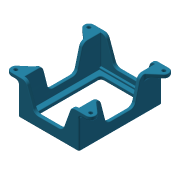
# Autodesk Inventor part: VatHolder
Saved by Autodesk Inventor 2014 (Build 180170000, 170)
## iProperties
Created: 2014-09-09
Part Number: VatHolder
Material: Generic
Document SubType Name: Modeling
Designer: Peele
Density: 1 g/cm^3
Appearance: Turquoise
Author: Peele
Autodesk Inventor part; units mm, degrees
ref_plane "YZ Plane" through (0, 0, 0) normal (1, 0, 0) x (0, 1, 0)
ref_plane "XZ Plane" through (0, 0, 0) normal (0, 1, 0) x (-1, 0, 0)
ref_plane "XY Plane" through (0, 0, 0) normal (0, 0, 1) x (1, 0, 0)
sketch "Sketch1" plane through (0, 0, 0) normal (0, 0, 1) x (1, 0, 0)
  line L0 (-38.1, -53.8) -> (38.1, -53.8)
  line L1 (38.1, -53.8) -> (38.1, 53.8)
  line L2 (38.1, 53.8) -> (-38.1, 53.8)
  line L3 (-38.1, 53.8) -> (-38.1, -53.8)
  line L4 (-38.1, -53.8) -> (38.1, 53.8) construction
  line L5 (38.1, -53.8) -> (-38.1, 53.8) construction
  line L6 (-30.6, -46.3) -> (30.6, -46.3)
  line L7 (30.6, -46.3) -> (30.6, 46.3)
  line L8 (30.6, 46.3) -> (-30.6, 46.3)
  line L9 (-30.6, 46.3) -> (-30.6, -46.3)
  line L10 (-30.6, -46.3) -> (30.6, 46.3) construction
  line L11 (30.6, -46.3) -> (-30.6, 46.3) construction
  line L12 (43.6, -59.3) -> (-43.6, -59.3)
  line L13 (-43.6, -59.3) -> (-43.6, 59.3)
  line L14 (-43.6, 59.3) -> (43.6, 59.3)
  line L15 (43.6, 59.3) -> (43.6, -59.3)
  line L16 (43.6, -59.3) -> (-43.6, 59.3) construction
  line L17 (-43.6, -59.3) -> (43.6, 59.3) construction
  point P0 (0, 0)
  dimension "d0" = 76.2
  dimension "d1" = 107.6
  dimension "d2" = 7.5
  dimension "d3" = 7.5
  dimension "d4" = 5.5
  dimension "d5" = 5.5
  constraints: 36 end point, 6 midpoint, 6 parallel, 3 horizontal, 3 perpendicular
  measures "d0" distance of L1.end L2.end
  measures "d1" distance of L0.end L1.end
  measures "d2" distance between parallel lines of L3 L9
  measures "d3" distance between parallel lines of L2 L8
  measures "d4" distance between parallel lines of L14 L2
  measures "d5" distance between parallel lines of L13 L3
extrude "Extrusion1" add sketch "Sketch1" along normal blind 5 contours L3 L2 L1 L0 | L12 L13 L14 L15
sketch "Sketch2" plane through (0, 0, 5) normal (0, 0, 1) x (1, 0, 0)
  line L0 (-43.6, 59.3) -> (-43.6, -59.3) projected
  line L1 (43.6, -59.3) -> (-43.6, -59.3)
  line L2 (-43.6, -59.3) -> (-43.6, 59.3)
  line L3 (-43.6, 59.3) -> (43.6, 59.3)
  line L4 (43.6, 59.3) -> (43.6, -59.3)
  line L5 (43.6, -59.3) -> (-43.6, 59.3) construction
  line L6 (-43.6, -59.3) -> (43.6, 59.3) construction
  line L7 (38.6, -54.3) -> (-38.6, -54.3)
  line L8 (-38.6, -54.3) -> (-38.6, 54.3)
  line L9 (-38.6, 54.3) -> (38.6, 54.3)
  line L10 (38.6, 54.3) -> (38.6, -54.3)
  line L11 (38.6, -54.3) -> (-38.6, 54.3) construction
  line L12 (-38.6, -54.3) -> (38.6, 54.3) construction
  point P0 (0, 0)
  dimension "d8" = 5
  dimension "d9" = 5
  constraints: 24 end point, 4 midpoint, 4 parallel, 2 horizontal, 2 perpendicular
  measures "d8" distance between parallel lines of L3 L9
  measures "d9" distance between parallel lines of L0 L8
extrude "Extrusion2" add sketch "Sketch2" along normal blind 45
sketch "Sketch3" plane through (-43.6, -59.3, 0) normal (0, -1, 0) x (1, 0, 0)
  line L0 (87.2, 0) -> (0, 0) projected
  line L1 (0, 50) -> (87.2, 50) projected
  line L2 (0, 0) -> (0, 50) projected
  line L3 (11.1, 50) -> (23.6, 15)
  line L4 (23.6, 15) -> (63.6, 15)
  line L5 (63.6, 15) -> (76.1, 50)
  line L6 (11.1, 50) -> (76.1, 50)
  line L7 (43.6, 0) -> (43.6, 15) construction
  dimension "d12" = 40
  dimension "d13" = 15
  dimension "d14" = 65
  constraints: 10 end point, 2 point on line, 1 collinear, 1 equal length, 1 midpoint, 1 perpendicular, 1 vertical
  measures "d12" distance of L3.end L4.end
  measures "d13" distance between parallel lines of L0 L4
  measures "d14" distance of L5.end L3.start
extrude "Extrusion3" cut sketch "Sketch3" against normal through all
sketch "Sketch4" plane through (0, 0, 50) normal (0, 0, 1) x (1, 0, 0)
  line L0 (43.6, -59.3) -> (43.6, 59.3) projected
  line L1 (43.6, -59.3) -> (43.6, -34.3)
  line L2 (43.6, -59.3) -> (53.6, -59.3)
  line L3 (58.199, -47.0228) -> (43.6, -34.3)
  arc A0 (53.6, -59.3) -> (58.199, -47.0228) centre (53.6, -52.3) ccw
  circle A1 centre (53.6, -52.3) radius 2.25
  point P0 (0, 0)
  dimension "d17" = 4.5
  dimension "d18" = 10
  dimension "d19" = 7
  dimension "d20" = 25
  constraints: 6 end point, 2 centre point, 2 point on circle, 2 tangent, 1 coincident, 1 perpendicular, 1 point on line
  measures "d17" diameter of A1
  measures "d18" distance from line of A0.centre L0
  measures "d19" distance from line of A0.centre L2
  measures "d20" distance from line of L1.end L2
extrude "Extrusion4" add sketch "Sketch4" against normal blind 6
mirror "Mirror1" about plane through (0, 0, 0) normal (0, 1, 0) of "Extrusion4"
mirror "Mirror2" about plane through (0, 0, 0) normal (1, 0, 0) of "Extrusion4", "Mirror1"
sketch "Sketch5" plane through (43.6, -59.3, 0) normal (1, 0, 0) x (0, 0, -1)
  line L0 (0, 118.6) -> (-44, 118.6) projected
  line L1 (-15, 79.3) -> (-15, 39.3)
  line L2 (-50, 93.6) -> (-50, 25)
  line L3 (-15, 39.3) -> (-50, 30.3)
  line L4 (-15, 79.3) -> (-50, 88.3)
  line L5 (-50, 30.3) -> (-50, 88.3)
  line L6 (0, 0) -> (-15, 39.3) construction
  line L7 (-15, 79.3) -> (0, 118.6) construction
  point P0 (0, 59.3)
  point P1 (-15, 118.6)
  dimension "d23" = 40
  dimension "d24" = 58
  constraints: 14 end point, 3 point on line, 2 equal length, 1 collinear, 1 perpendicular
  measures "d23" distance of L1.end L1.start
  measures "d24" distance of L3.end L4.end
extrude "Extrusion5" cut sketch "Sketch5" against normal through all
sketch "Sketch6" plane through (0, 0, 5) normal (0, 0, 1) x (1, 0, 0)
  line L0 (-38.6, 54.3) -> (-38.6, -54.3) projected
  line L1 (-38.6, -54.3) -> (38.6, -54.3) projected
  line L2 (38.6, -54.3) -> (38.6, 54.3) projected
  line L3 (-38.6, 54.3) -> (38.6, 54.3)
  line L4 (38.6, 54.3) -> (38.6, 51.8)
  line L5 (38.6, 51.8) -> (-38.6, 51.8)
  line L6 (-38.6, 51.8) -> (-38.6, 54.3)
  line L7 (38.6, -54.3) -> (-38.6, -54.3)
  line L8 (-38.6, -54.3) -> (-38.6, -51.8)
  line L9 (-38.6, -51.8) -> (38.6, -51.8)
  line L10 (38.6, -51.8) -> (38.6, -54.3)
  point P0 (0, 0)
  dimension "d27" = 2.5
  dimension "d28" = 2.5
  constraints: 16 end point, 4 parallel, 2 horizontal, 2 perpendicular, 2 point on line
  measures "d27" distance of L5.end L0.start
  measures "d28" distance between parallel lines of L1 L9
extrude "Extrusion6" add sketch "Sketch6" along normal blind 2.9 contours L3 L2 L5 L0 | L9 L2 L1 L0
fillet "Fillet1" radius 8 16 edges at (-20, -56.8, 15) (-32.5, -56.8, 50) (-41.1, -29, 50) (-41.1, -20, 15) (-41.1, 29, 50) (-41.1, 20, 15) (-20, 56.8, 15) (-32.5, 56.8, 50) (20, 56.8, 15) (32.5, 56.8, 50) (41.1, 29, 50) (41.1, 20, 15) (20, -56.8, 15) (32.5, -56.8, 50) (41.1, -29, 50) (41.1, -20, 15)
fillet "Fillet2" radius 4 12 edges at (-43.6, -46.8, 44) (-43.6, -34.3, 46.9744) (-43.6, 46.8, 44) (-43.6, 34.3, 46.9744) (30.6, 46.3, 2.5) (-30.6, 46.3, 2.5) (-30.6, -46.3, 2.5) (30.6, -46.3, 2.5) (43.6, -34.3, 46.9744) (43.6, -46.8, 44) (43.6, 46.8, 44) (43.6, 34.3, 46.9744)
fillet "Fillet3" radius 1 18 edges at (0, -51.8, 7.9) (-29.4284, -45.1284, 5) (-30.6, 0, 5) (-29.4284, 45.1284, 5) (0, 46.3, 5) (29.4284, 45.1284, 5) (30.6, 0, 5) (29.4284, -45.1284, 5) (0, -46.3, 5) (29.4284, -45.1284, 0) (30.6, 0, 0) (29.4284, 45.1284, 0) (0, 46.3, 0) (-29.4284, 45.1284, 0) (-30.6, 0, 0) (-29.4284, -45.1284, 0) (0, -46.3, 0) (0, 51.8, 7.9)
fillet "Fillet4" radius 1 36 edges at (38.6, -30.301, 48.3221) (38.6, -24.5, 32.5) (38.6, -18.699, 16.6779) (38.6, 0, 15) (38.6, 18.699, 16.6779) (38.6, 24.5, 32.5) (38.6, 30.301, 48.3221) (38.6, 44.7516, 50) (38.6, -44.7516, 50) (26.25, -54.3, 32.5) (18.9706, -54.3, 16.4607) (0, -54.3, 15) (-18.9706, -54.3, 16.4607) (-26.25, -54.3, 32.5) (-33.5294, -54.3, 48.5393) (-38.3689, -54.3, 50) (38.3689, -54.3, 50) (33.5294, -54.3, 48.5393) (38.3689, 54.3, 50) (26.25, 54.3, 32.5) (18.9706, 54.3, 16.4607) (0, 54.3, 15) (-18.9706, 54.3, 16.4607) (-26.25, 54.3, 32.5) (-33.5294, 54.3, 48.5393) (-38.3689, 54.3, 50) (33.5294, 54.3, 48.5393) (-38.6, 30.301, 48.3221) (-38.6, 24.5, 32.5) (-38.6, 18.699, 16.6779) (-38.6, 0, 15) (-38.6, -18.699, 16.6779) (-38.6, -24.5, 32.5) (-38.6, -30.301, 48.3221) (-38.6, -44.7516, 50) (-38.6, 44.7516, 50)
fillet "Fillet5" radius 1 48 edges at (60.1552, 54.7555, 50) (51.5855, 41.2592, 50) (44.8171, 35.3534, 50) (43.8895, 33.9741, 49.905) (43.6, 29.2824, 47.38) (43.6, 24.5, 32.5) (43.6, 18.699, 16.6779) (43.6, 0, 15) (43.6, -18.699, 16.6779) (43.6, -24.5, 32.5) (43.6, -29.2824, 47.38) (43.8895, -33.9741, 49.905) (44.8171, -35.3534, 50) (51.5855, -41.2592, 50) (60.1552, -54.7555, 50) (45.8689, -59.3, 50) (33.5294, -59.3, 48.5393) (26.25, -59.3, 32.5) (18.9706, -59.3, 16.4607) (0, -59.3, 15) (-18.9706, -59.3, 16.4607) (-26.25, -59.3, 32.5) (-33.5294, -59.3, 48.5393) (-45.8689, -59.3, 50) (-60.1552, -54.7555, 50) (-51.5855, -41.2592, 50) (-44.8171, -35.3534, 50) (-43.8895, -33.9741, 49.905) (-43.6, -29.2824, 47.38) (-43.6, -24.5, 32.5) (-43.6, -18.699, 16.6779) (-43.6, 0, 15) (-43.6, 18.699, 16.6779) (-43.6, 24.5, 32.5) (-43.6, 29.2824, 47.38) (-43.8895, 33.9741, 49.905) (-44.8171, 35.3534, 50) (-51.5855, 41.2592, 50) (-60.1552, 54.7555, 50) (-45.8689, 59.3, 50) (-33.5294, 59.3, 48.5393) (-26.25, 59.3, 32.5) (-18.9706, 59.3, 16.4607) (0, 59.3, 15) (18.9706, 59.3, 16.4607) (26.25, 59.3, 32.5) (33.5294, 59.3, 48.5393) (45.8689, 59.3, 50)
fillet "Fillet6" radius 2 28 edges at (44.7716, 59.3, 42.8284) (50.6, 59.3, 44) (60.1552, 54.7555, 44) (52.8995, 42.4044, 44) (46.1968, 36.5631, 43.7458) (43.9591, 34.1366, 41.6565) (43.6, 59.3, 20) (44.7716, -59.3, 42.8284) (50.6, -59.3, 44) (60.1552, -54.7555, 44) (52.8995, -42.4044, 44) (46.1968, -36.5631, 43.7458) (43.9591, -34.1366, 41.6565) (43.6, -59.3, 20) (-44.7716, -59.3, 42.8284) (-50.6, -59.3, 44) (-60.1552, -54.7555, 44) (-52.8995, -42.4044, 44) (-46.1968, -36.5631, 43.7458) (-43.9591, -34.1366, 41.6565) (-43.6, -59.3, 20) (-44.7716, 59.3, 42.8284) (-50.6, 59.3, 44) (-60.1552, 54.7555, 44) (-52.8995, 42.4044, 44) (-46.1968, 36.5631, 43.7458) (-43.9591, 34.1366, 41.6565) (-43.6, 59.3, 20)
fillet "Fillet7" radius 1 16 edges at (-43.0142, 58.7142, 0) (0, 59.3, 0) (43.0142, 58.7142, 0) (43.6, 0, 0) (43.0142, -58.7142, 0) (0, -59.3, 0) (-43.0142, -58.7142, 0) (-43.6, 0, 0) (51.35, 52.3, 50) (51.35, -52.3, 50) (-51.35, -52.3, 50) (-51.35, 52.3, 50) (-51.35, 52.3, 44) (-51.35, -52.3, 44) (51.35, 52.3, 44) (51.35, -52.3, 44)
fillet "Fillet8" radius 0.5 26 edges at (38.8929, 54.5929, 49.7071) (38.6, 54.3, 28.45) (38.6, 0, 5) (38.6, 53.55, 7.9) (38.6, 51.8, 5.95) (38.6, 52.0929, 7.6071) (0, 54.3, 7.9) (0, 51.8, 5) (38.8929, -54.5929, 49.7071) (38.6, -54.3, 28.45) (38.6, -51.8, 5.95) (38.6, -53.55, 7.9) (38.6, -52.0929, 7.6071) (0, -54.3, 7.9) (0, -51.8, 5) (-38.6, -53.55, 7.9) (-38.6, -51.8, 5.95) (-38.6, -52.0929, 7.6071) (-38.8929, -54.5929, 49.7071) (-38.6, -54.3, 28.45) (-38.6, 0, 5) (-38.6, 52.0929, 7.6071) (-38.6, 53.55, 7.9) (-38.6, 51.8, 5.95) (-38.8929, 54.5929, 49.7071) (-38.6, 54.3, 28.45)
equation "\"d3\" = d2"
equation "\"d5\" = d4"
equation "\"d8\" = d9"
equation "\"d28\" = d27"
body "Solid1"
